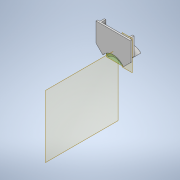
# Autodesk Inventor part: CTF_deksel
Saved by Autodesk Inventor 2020.5 (Build 245400000, 400)
## iProperties
Created: 2022-03-21
Part Number: CTF_deksel
Material: Generic
Document SubType Name: Modeling
Designer: EDDY
Density: 1 g/cm^3
Appearance: Default
Author: EDDY
Autodesk Inventor part; units mm, degrees
ref_plane "YZ Plane" through (0, 0, 0) normal (1, 0, 0) x (0, 1, 0)
ref_plane "XZ Plane" through (0, 0, 0) normal (0, 1, 0) x (-1, 0, 0)
ref_plane "XY Plane" through (0, 0, 0) normal (0, 0, 1) x (1, 0, 0)
ref_plane "Work Plane1" through (0, 0, 0) normal (0, 0, 1) x (1, 0, 0)
sketch "Sketch1" plane through (0, 0, 0) normal (0, 0, 1) x (1, 0, 0)
  line L0 (-31, 62.928932) -> (-27, 62.928932)
  line L1 (27, 62.928932) -> (31, 62.928932)
  line L2 (31, 28.272078) -> (16.684834, 13.956912)
  line L3 (14.142136, 17.071068) -> (27, 29.928933)
  circle A0 centre (0, 2.928932) radius 22.6
  line L4 (-27, 29.928933) -> (-14.142136, 17.071068)
  line L5 (-16.684834, 13.956912) -> (-31, 28.272078)
  line L6 (-31, 28.272078) -> (-31, 62.928932)
  line L7 (-27, 62.928932) -> (-27, 29.928933)
  line L8 (27, 29.928933) -> (27, 62.928932)
  circle A1 centre (0, 2.928932) radius 20.2
  line L9 (-31, 62.928932) -> (31, 62.928932)
  line L10 (31, 62.928932) -> (31, 28.272078)
  line L11 (31, 28.272078) -> (16.684834, 13.956912)
  point P0 (0, 0)
  point P1 (-18.556746, 15.828823)
  point P2 (18.556746, 15.828823)
  constraints: 2 end point, 1 horizontal
sketch "Sketch1 outline for Extrusion1" plane through (0, 0, 0) normal (0, 0, 1) x (1, 0, 0)
  line L0 (27, 62.928932) -> (-27, 62.928932)
  line L1 (31, 62.928932) -> (27, 62.928932)
  line L2 (31, 28.272078) -> (31, 62.928932)
  line L3 (18.556746, 15.828823) -> (31, 28.272078)
  arc A0 (-18.556746, 15.828823) -> (18.556746, 15.828823) centre (0, 2.928932) cw
  line L4 (-31, 28.272078) -> (-18.556746, 15.828823)
  line L5 (-31, 62.928932) -> (-31, 28.272078)
  line L6 (-27, 62.928932) -> (-31, 62.928932)
extrude "Extrusion1" add sketch "Sketch1 outline for Extrusion1" along normal blind 3
sketch "Sketch2" plane through (0, 0, 0) normal (0, 0, -1) x (-1, 0, 0)
  line L0 (-27, 29.928933) -> (-27, 62.928932)
  line L1 (-14.142136, 17.071068) -> (-27, 29.928933)
  line L2 (27, 29.928933) -> (14.142136, 17.071068)
  circle A0 centre (0, 2.928932) radius 22.6
  line L3 (27, 62.928932) -> (27, 29.928933)
  line L4 (-31, 62.928932) -> (31, 62.928932)
  line L5 (-27, 29.928933) -> (-27, 62.928932)
  line L6 (-9.710839, 16.882412) -> (-24, 31.171573)
  line L7 (-24, 31.171573) -> (-24, 62.928932)
  line L8 (27, 29.928933) -> (14.142136, 17.071068)
  line L9 (27, 62.928932) -> (27, 29.928933)
  line L10 (24, 62.928932) -> (24, 31.171573)
  line L11 (24, 31.171573) -> (9.710839, 16.882412)
  arc A1 (13.219381, 13.617616) -> (-13.219381, 13.617616) centre (0, 2.928932) ccw
  line L12 (-27, 29.928933) -> (-12.020815, 14.949747)
  line L13 (27.001712, 29.930644) -> (12.020815, 14.949747)
  line L14 (27, 62.928932) -> (24, 62.928932)
  circle A2 centre (0, 2.928932) radius 16.505526
  point P0 (0, 0)
  dimension "d2" = 3
  dimension "d3" = 3
  dimension "d4" = 3
  dimension "d5" = 3
  constraints: 14 end point, 4 parallel, 4 point on circle, 3 collinear, 2 point on line, 1 vertical
  measures "d2" distance between parallel lines of L7 L0
  measures "d3" distance between parallel lines of L3 L10
  measures "d4" distance between parallel lines of L2 L11
  measures "d5" distance between parallel lines of L6 L1
sketch "Sketch2 outline for Extrusion2" plane through (0, 0, 0) normal (0, 0, -1) x (-1, 0, 0)
  line L0 (24, 31.171573) -> (9.710839, 16.882412)
  arc A0 (9.710839, 16.882412) -> (12.020815, 14.949747) centre (0, 2.928932) cw
  line L1 (12.020815, 14.949747) -> (27, 29.928933)
  line L2 (27, 29.928933) -> (27, 62.928932)
  line L3 (27, 62.928932) -> (24, 62.928932)
  line L4 (24, 62.928932) -> (24, 31.171573)
  line L5 (-24, 31.171573) -> (-24, 62.928932)
  line L6 (-24, 62.928932) -> (-27, 62.928932)
  line L7 (-27, 62.928932) -> (-27, 29.928933)
  line L8 (-27, 29.928933) -> (-12.020815, 14.949747)
  arc A1 (-12.020815, 14.949747) -> (-9.710839, 16.882412) centre (0, 2.928932) cw
  line L9 (-9.710839, 16.882412) -> (-24, 31.171573)
extrude "Extrusion2" add sketch "Sketch2 outline for Extrusion2" along normal blind 8
ref_plane "Work Plane2" through (0, 2.928932, 0) normal (0, 0, -1) x (-1, 0, 0)
ref_plane "Work Plane3" through (0, 2.928932, 0) normal (0, 0, -1) x (-1, 0, 0)
thicken "Thicken1" operation add thickness 0.3 both sides no extend neighbours yes toward (-0.6930325, -0.7209063, 0) faces at (11.781552, 15.18434, -2.666667) (-9.983973, 16.688303, -2.666667)
ref_plane "Work Plane4" through (0, 2.928932, 88.5) normal (1, 0, 0) x (0, 1, 0)
sketch "Sketch5" plane through (0, 2.928932, 88.5) normal (1, 0, 0) x (0, 1, 0)
  line L0 (16.8, -88.5) -> (16.8, -123.5)
  line L1 (16.8, -123.5) -> (20.338452, -121.457074)
  line L2 (20.338452, -121.457074) -> (35.706588, -88.5)
  line L3 (35.706588, -88.5) -> (16.8, -88.5)
  line L4 (17.960512, -88.5) -> (28.242641, -88.5)
  line L5 (72.585786, -88.5) -> (-15.514719, -88.5)
  line L6 (16.5, 82.1) -> (16.5, -191.6)
  line L7 (-2.15, -148.5) -> (-2.15, 1.5)
  line L8 (0, -191.6) -> (0, 82.1)
  point P0 (-2.928932, -88.5)
  dimension "d24" = 0.3
  dimension "d25" = 35
  dimension "d26" = 60
  dimension "d27" = 25
  constraints: 14 end point, 4 vertical, 2 point on line, 1 collinear, 6 other
  measures "d24" distance between parallel lines of L6 L0
  measures "d25" distance of L0.start L0.end
  measures "d26" angle of L0 L1
  measures "d27" angle of L0 L2
sketch "Sketch5 outline for Revolution1" plane through (0, 2.928932, 88.5) normal (1, 0, 0) x (0, 1, 0)
  line L0 (16.8, -123.5) -> (20.338452, -121.457074)
  line L1 (16.8, -88.5) -> (16.8, -123.5)
  line L2 (35.706588, -88.5) -> (16.8, -88.5)
  line L3 (20.338452, -121.457074) -> (35.706588, -88.5)
revolve "Revolution1" add sketch "Sketch5 outline for Revolution1" angle 90 mid plane about axis through (0, 2.928932, -103.1) along (0, 0, 1)
fillet "Fillet2" radius 5 3 edges at (21.6771, 28.8487, -4.1112) (0, 38.6355, 0) (-21.6771, 28.8487, -4.1112)
fillet "Fillet4" radius 2 2 edges at (27, 29.9289, -4) (-27, 29.9289, -4)
body "Solid1"
